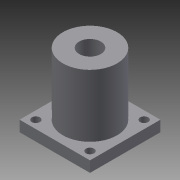
# Autodesk Inventor part: Flange Mount Linear Bearing (McMaster Part #64825K11)
Saved by Autodesk Inventor 2014 SP1 (Build 180222100, 222)
## iProperties
Created: 2014-01-06
Part Number: Flange Mount Linear Bearing (McMaster Part #64825K11)
Material: Generic
Document SubType Name: Modeling
Designer: Andrew Toennies
Density: 1 g/cm^3
Appearance: Default
Mass: 33.8439 g
Surface Area: 97.919 cm^2
Volume: 33.8439 cm^3
Author: Andrew Toennies
Autodesk Inventor part; units mm, degrees
ref_plane "YZ Plane" through (0, 0, 0) normal (1, 0, 0) x (0, 1, 0)
ref_plane "XZ Plane" through (0, 0, 0) normal (0, 1, 0) x (-1, 0, 0)
ref_plane "XY Plane" through (0, 0, 0) normal (0, 0, 1) x (1, 0, 0)
sketch "Sketch1" plane through (0, 0, 0) normal (0, 1, 0) x (-1, 0, 0)
  line L0 (0, 0) -> (-41.275, 0)
  line L1 (-41.275, 0) -> (-41.275, 41.275)
  line L2 (-41.275, 41.275) -> (0, 41.275)
  line L3 (0, 41.275) -> (0, 0)
  circle A0 centre (-20.6375, 20.6375) radius 6.35
  line L4 (0, 41.275) -> (-41.275, 0) construction
  line L5 (-41.275, 41.275) -> (0, 0) construction
  dimension "d0" = 41.275
  dimension "d1" = 41.275
  dimension "d15" = 12.7
  constraints: 12 end point, 2 midpoint, 2 parallel, 1 centre point, 1 horizontal, 1 perpendicular
  measures "d0" distance of L1.end L2.end
  measures "d1" distance of L2.end L0.start
  measures "d15" diameter of A0
extrude "Extrusion1" add sketch "Sketch1" along normal blind 6.35
sketch "Sketch2" plane through (0, 6.35, 0) normal (0, 1, 0) x (1, 0, 0)
  circle A0 centre (20.6375, -20.6375) radius 6.35
  circle A1 centre (20.6375, -20.6375) radius 15.875
  dimension "d4" = 12.7
  dimension "d5" = 31.75
  constraints: 2 centre point, 1 coincident
  measures "d4" diameter of A0
  measures "d5" diameter of A1
extrude "Extrusion2" add sketch "Sketch2" along normal blind 36.5125
sketch "Sketch3" plane through (0, 6.35, 0) normal (0, 1, 0) x (1, 0, 0)
  line L0 (0, -41.275) -> (41.275, -41.275) projected
  line L1 (41.275, -41.275) -> (41.275, 0) projected
  circle A0 centre (20.6375, -20.6375) radius 15.875 projected
  circle A1 centre (4.7625, -4.7625) radius 2.3813
  circle A2 centre (36.5125, -4.7625) radius 2.3813
  circle A3 centre (36.5125, -36.5125) radius 2.3813
  circle A4 centre (4.7625, -36.5125) radius 2.3813
  line L2 (4.7625, -36.5125) -> (4.7625, -4.7625) construction
  line L3 (4.7625, -4.7625) -> (36.5125, -4.7625) construction
  line L4 (36.5125, -4.7625) -> (36.5125, -36.5125) construction
  line L5 (36.5125, -36.5125) -> (4.7625, -36.5125) construction
  dimension "d8" = 4.7625
  dimension "d10" = 31.75
  dimension "d11" = 15.875
  dimension "d12" = 15.875
  constraints: 8 end point, 4 centre point, 3 equal radius, 3 perpendicular, 2 parallel
  measures "d8" diameter of A2
  measures "d10" distance of L2.end L3.end
  measures "d11" distance from line of L4 A0.centre
  measures "d12" distance from line of A0.centre L3
extrude "Extrusion3" cut sketch "Sketch3" against normal blind 36.5125 contours A1 | A2 | A3 | A4
body "Solid1"
